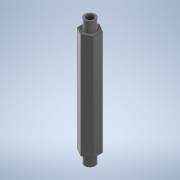
# Autodesk Inventor part: PlanetShaft
Saved by Autodesk Inventor 2020 (Build 240168000, 168)
## iProperties
Created: 2019-06-07
Part Number: PlanetShaft
Material: Aluminum 6061
Document SubType Name: Modeling
Designer: Connor
Density: 2.7 g/cm^3
Appearance: Smooth - Black
Mass: 13.3392 g
Surface Area: 22.9538 cm^2
Volume: 4.94045 cm^3
Author: Connor
Autodesk Inventor part; units mm, degrees
ref_plane "YZ Plane" through (0, 0, 0) normal (1, 0, 0) x (0, 1, 0)
ref_plane "XZ Plane" through (0, 0, 0) normal (0, 1, 0) x (-1, 0, 0)
ref_plane "XY Plane" through (0, 0, 0) normal (0, 0, 1) x (1, 0, 0)
sketch "Sketch1" plane through (0, 0, 0) normal (0, 1, 0) x (-1, 0, 0)
  line L0 (0, -5.4993) -> (-4.7625, -2.7496)
  line L1 (-4.7625, -2.7496) -> (-4.7625, 2.7496)
  line L2 (-4.7625, 2.7496) -> (0, 5.4993)
  line L3 (0, 5.4993) -> (4.7625, 2.7496)
  line L4 (4.7625, 2.7496) -> (4.7625, -2.7496)
  line L5 (4.7625, -2.7496) -> (0, -5.4993)
  circle A0 centre (0, 0) radius 2.0955
  dimension "d0" = 9.525
  dimension "d9" = 4.191
  constraints: 12 end point, 2 coincident, 1 centre point, 1 vertical alignment, 13 other
  measures "d0" distance between parallel lines of L1 L4
  measures "d9" diameter of A0
extrude "Extrusion1" add sketch "Sketch1" along normal blind 76.2
sketch "Sketch2" plane through (0, 76.2, 0) normal (0, 1, 0) x (1, 0, 0)
  circle A0 centre (0, 0) radius 3.175
  line L0 (-4.7625, 2.7496) -> (-4.7625, -2.7496) projected
  line L1 (-4.7625, -2.7496) -> (0, -5.4993) projected
  line L2 (0, -5.4993) -> (4.7625, -2.7496) projected
  line L3 (4.7625, -2.7496) -> (4.7625, 2.7496) projected
  line L4 (4.7625, 2.7496) -> (0, 5.4993) projected
  line L5 (0, 5.4993) -> (-4.7625, 2.7496) projected
  dimension "d3" = 6.35
  constraints: 1 centre point, 1 coincident
  measures "d3" diameter of A0
extrude "Extrusion2" cut sketch "Sketch2" against normal blind 6.35
sketch "Sketch3" plane through (0, 0, 0) normal (0, -1, 0) x (1, 0, 0)
  circle A0 centre (0, 0) radius 3.175
  line L0 (-4.7625, -2.7496) -> (-4.7625, 2.7496) projected
  line L1 (0, -5.4993) -> (-4.7625, -2.7496) projected
  line L2 (4.7625, -2.7496) -> (0, -5.4993) projected
  line L3 (4.7625, 2.7496) -> (4.7625, -2.7496) projected
  line L4 (0, 5.4993) -> (4.7625, 2.7496) projected
  line L5 (-4.7625, 2.7496) -> (0, 5.4993) projected
  dimension "d6" = 6.35
  constraints: 1 centre point, 1 coincident
  measures "d6" diameter of A0
extrude "Extrusion3" cut sketch "Sketch3" against normal blind 6.35
body "Solid1"
